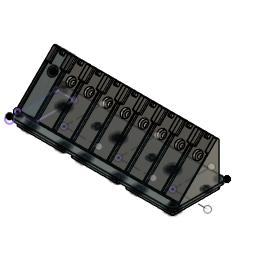
holder_v1 (Autodesk Fusion 360 design; units mm, degrees)
Autodesk Fusion 360 part; units mm, degrees
ref_plane "WorkPlane1" through (12.125, 0, 0) normal (0, -0.707107, 0.707107) x (1, 0, 0) in component "blade_holder"
sketch "Sketch1" plane through (0, 0, 0) normal (0, -0.707107, 0.707107) x (1, 0, 0) in component "blade_holder"
  line L0 (0, 42) -> (14, 42)
  line L1 (14, 42) -> (14, 0)
  line L2 (14, 0) -> (0, 0)
  line L3 (0, 0) -> (0, 42)
  line L4 (1, 41) -> (13, 41)
  line L5 (13, 41) -> (13, 1)
  line L6 (13, 1) -> (1, 1)
  line L7 (1, 1) -> (1, 41)
  line L8 (1, 41) -> (1, 42)
  line L9 (13, 41) -> (13, 42)
  line L10 (6, 42) -> (8, 42)
  line L11 (8, 42) -> (8, 39)
  line L12 (8, 39) -> (6, 39)
  line L13 (6, 39) -> (6, 42)
  line L14 (3, 42) -> (3, 32)
  line L15 (3, 32) -> (1, 32)
  line L16 (11, 42) -> (11, 32)
  line L17 (11, 32) -> (13, 32)
  line L18 (3, 32) -> (11, 32) construction
  circle A0 centre (7, 28.75) radius 3.25
  circle A1 centre (7, 28.75) radius 1.625
  dimension "d7" = 14
  dimension "d8" = 42
  dimension "d9" = 12
  dimension "d10" = 40
  dimension "d11" = 1
  dimension "d12" = 1
  dimension "d14" = 1
  dimension "d15" = 1
  dimension "d22" = 2
  dimension "d23" = 3
  dimension "d24" = 3
  dimension "d25" = 6
  dimension "d40" = 2
  dimension "d41" = 2
  dimension "d42" = 10
  dimension "d43" = 10
  dimension "d116" = 6.5
  dimension "d117" = 6
  dimension "d125" = 3.25
  constraint horizontal L0
  constraint vertical L1
  constraint horizontal L2
  constraint vertical L3
  constraint horizontal L4
  constraint vertical L5
  constraint horizontal L6
  constraint vertical L7
  constraint coincident L0 L8.end
  constraint perpendicular L0 L8
  constraint coincident L0 L9.end
  constraint perpendicular L0 L9
  constraint horizontal L10
  constraint vertical L11
  constraint horizontal L12
  constraint vertical L13
  constraint coincident L0 L14.start
  constraint perpendicular L4 L14
  constraint coincident L7 L15.end
  constraint perpendicular L7 L15
  constraint coincident L0 L16.start
  constraint perpendicular L4 L16
  constraint coincident L5 L17.end
  constraint perpendicular L5 L17
  constraint tangent L18 A0
  constraint concentric A0 A1
  measures "d7" distance of L0.start L0.end
  measures "d8" distance of L0.end L1.end
  measures "d9" distance of L4.start L4.end
  measures "d10" distance of L4.start L6.end
  measures "d11" distance of L0 L4
  measures "d12" distance of L1 L5
  measures "d14" distance of L2.end L6
  measures "d15" distance of L2.end L7
  measures "d22" distance of L10.start L10.end
  measures "d23" distance of L10.end L11.end
  measures "d24" distance of L0 L12
  measures "d25" distance of L3 L13
  measures "d40" distance of L14.end L15.end
  measures "d41" distance of L16.end L17.end
  measures "d42" distance of L16.start L16.end
  measures "d43" distance of L14.start L14.end
  measures "d116" diameter of A0
  measures "d117" distance of L7 A0.centre
  measures "d125" diameter of A1
sketch "Sketch2" plane through (0, 0, 0) normal (0, 0, 1) x (1, 0, 0) in component "blade_holder"
  line L0 (0, 0) -> (0, 29.6985)
  line L1 (0, 29.6985) -> (14, 29.6985)
  line L2 (14, 29.6985) -> (14, 0)
  line L3 (14, 0) -> (0, 0)
sketch "Sketch3" plane through (0, 0, 0) normal (0, 0, 1) x (1, 0, 0) in component "blade_holder"
  line L0 (3.75, 35.8492) -> (122.25, 35.8492)
  line L1 (126, 32.0992) -> (126, -2.4008)
  line L2 (122.25, -6.1508) -> (3.75, -6.1508)
  line L3 (0, -2.4008) -> (0, 32.0992)
  arc A0 (3.75, 35.8492) -> (0, 32.0992) centre (3.75, 32.0992) ccw
  arc A1 (126, 32.0992) -> (122.25, 35.8492) centre (122.25, 32.0992) ccw
  arc A2 (122.25, -6.1508) -> (126, -2.4008) centre (122.25, -2.4008) ccw
  arc A3 (0, -2.4008) -> (3.75, -6.1508) centre (3.75, -2.4008) ccw
  point P0 (0, 35.8492)
  point P1 (126, 35.8492)
  point P2 (0, -6.1508)
  dimension "d91" = 126
  dimension "d92" = 42
  dimension "d93" = 6.1508
  dimension "d95" = 126
  dimension "d96" = 3.75
  dimension "d97" = 3.75
  dimension "d98" = 3.75
  dimension "d99" = 3.75
  constraint horizontal L0
  constraint vertical L1
  constraint horizontal L2
  constraint vertical L3
  constraint coincident P0 L0
  constraint coincident P0 L3
  constraint tangent L0 A0
  constraint tangent L3 A0
  constraint coincident P1 L0
  constraint coincident P1 L1
  constraint tangent L0 A1
  constraint tangent L1 A1
  constraint tangent L1 A2
  constraint tangent L2 A2
  constraint coincident P2 L3
  constraint coincident P2 L2
  constraint tangent L3 A3
  constraint tangent L2 A3
  measures "d91" distance of P0 P1
  measures "d92" distance of P0 P2
  measures "d93" distance of origin L2
  measures "d95" distance of origin L1
  measures "d96" radius of A0
  measures "d97" radius of A1
  measures "d98" radius of A2
  measures "d99" radius of A3
extrude "Extrude1" add sketch "Sketch1" along normal blind 2 contours L0 L1 L2 L3 L5 L6 L7 L8 L9 | L0 L4 L8 L14 | L4 L7 L14 L15 | L0 L4 L9 L16 | L4 L5 L16 L17 makes body 1 in component "blade_holder"
extrude "Extrude2" add sketch "Sketch2" along normal up to surface end surface through (12.125, 0, 0) normal (0, -0.707107, 0.707107) offset 0 bodies 1 in component "blade_holder"
extrude "Extrude3" add sketch "Sketch1" along normal blind 3 contours L0 L4 L10 L11 L13 | L4 L11 L12 L13 bodies 1 in component "blade_holder"
extrude "Extrude7" cut sketch "Sketch1" against normal blind 2.5 contours A0 | A1 bodies 1 in component "blade_holder"
extrude "Extrude8" cut sketch "Sketch1" against normal blind 5 contours A1 bodies 1 in component "blade_holder"
fillet "Fillet1" radius 0.5 8 edges at (6, 28.6378, 30.7591) (6, 26.5165, 30.7591) (7, 27.5772, 31.8198) (8, 28.6378, 30.7591) (8, 26.5165, 30.7591) (7, 25.4558, 29.6985) (8, 26.5165, 28.6378) (6, 26.5165, 28.6378) on bodies 1 in component "blade_holder"
fillet "Fillet1" radius 0.5 17 edges at (3, 28.9914, 30.4056) (3, 21.9203, 23.3345) (1, 10.253, 13.0815) (2, 21.2132, 24.0416) (3, 24.7487, 27.5772) (7, -0.7071, 2.1213) (1, 0, 1.4142) (11, 28.9914, 30.4056) (11, 21.9203, 23.3345) (12, 21.2132, 24.0416) (13, 10.253, 13.0815) (13, 0, 1.4142) (1, 21.9203, 23.3345) (13, 21.9203, 23.3345) (11, 24.7487, 27.5772) (12.5, 28.2843, 31.1127) (1.5, 28.2843, 31.1127) on bodies 1 in component "blade_holder"
extrude "Extrude6" add sketch "Sketch3" against normal blind 2 separate body makes body 2 in component "blade_holder"
sketch "Sketch4" plane through (0, 0, -2) normal (0, 0, -1) x (1, 0, 0) in component "blade_holder"
  arc A0 (0, -32.0992) -> (3.75, -35.8492) centre (3.75, -32.0992) ccw
  line L0 (3.75, -35.8492) -> (122.25, -35.8492)
  arc A1 (122.25, -35.8492) -> (126, -32.0992) centre (122.25, -32.0992) ccw
  line L1 (126, -32.0992) -> (126, 2.4008)
  arc A2 (126, 2.4008) -> (122.25, 6.1508) centre (122.25, 2.4008) ccw
  line L2 (122.25, 6.1508) -> (3.75, 6.1508)
  arc A3 (3.75, 6.1508) -> (0, 2.4008) centre (3.75, 2.4008) ccw
  line L3 (0, 2.4008) -> (0, -32.0992)
  circle A4 centre (8, -1.8492) radius 2.5
  point P0 (0, 6.1508)
  dimension "d104" = 5
  dimension "d105" = 8
  dimension "d106" = 8
  measures "d104" diameter of A4
  measures "d105" vertical distance of A4.centre P0
  measures "d106" horizontal distance of A4.centre P0
pattern_linear "R-Pattern1" count 9 spacing 14 along (1, 0, 0) of bodies 1 makes body 3 at (14, 19.2097, 10.253) makes body 4 at (32.6667, 19.799, 0) makes body 5 at (51.3333, 9.8995, 0) makes body 6 at (60.6667, 19.799, 0) makes body 7 at (74.6667, 19.799, 0) makes body 8 at (88.6667, 19.799, 0) makes body 9 at (102.6667, 19.799, 0) makes body 10 at (126, 19.2097, 10.253) in component "blade_holder"
sketch "Sketch2 (2)" plane through (0, 0, 0) normal (0, 1, 0) x (1, 0, 0) in component "gridfinity_leg"
  line L0 (17.8, 0) -> (18.6, -0.8)
  line L1 (18.6, -0.8) -> (18.6, -2.6)
  line L2 (18.6, -2.6) -> (20.75, -4.75)
  line L3 (0, 0) -> (27.8, 0) construction
  line L4 (20.75, -4.75) -> (0, -4.75)
  line L5 (0, -4.75) -> (0, 0)
  line L6 (17.8, 0) -> (0, 0)
  line L7 (0, -4.75) -> (0, 0)
  dimension "d6_1" = 0.8
  dimension "d7_1" = 45
  dimension "d8_1" = 1.8
  dimension "d9_1" = 2.15
  dimension "d10_1" = 45
  dimension "d15_1" = 20.75
  dimension "d16_1" = 4.75
  constraint vertical L1
  constraint coincident L3.start L5.end
  constraint horizontal L3
  constraint coincident L0.start L3
  constraint perpendicular L3 L5
  measures "d6_1" horizontal distance of L0.start L0.end
  measures "d7_1" angle of L0 L3
  measures "d8_1" distance of L0.end L1.end
  measures "d9_1" horizontal distance of L1.end L2.end
  measures "d10_1" angle of L2 L3
  measures "d15_1" distance of L2.end L4.end
  measures "d16_1" distance of L4.end L3.start
sketch "Sketch4 (2)" plane through (0, 0, 0) normal (0, 0, 1) x (1, 0, 0) in component "gridfinity_leg"
  line L0 (-17, 20.75) -> (17, 20.75)
  line L1 (20.75, 17) -> (20.75, -17)
  line L2 (17, -20.75) -> (-17, -20.75)
  line L3 (-20.75, -17) -> (-20.75, 17)
  arc A0 (-17, 20.75) -> (-20.75, 17) centre (-17, 17) ccw
  arc A1 (20.75, 17) -> (17, 20.75) centre (17, 17) ccw
  arc A2 (17, -20.75) -> (20.75, -17) centre (17, -17) ccw
  arc A3 (-20.75, -17) -> (-17, -20.75) centre (-17, -17) ccw
  point P0 (-20.75, 20.75)
  point P1 (20.75, 20.75)
  point P2 (20.75, -20.75)
  dimension "d43_1" = 41.5
  dimension "d44_1" = 41.5
  dimension "d45_1" = 20.75
  dimension "d46_1" = 20.75
  dimension "d47_1" = 3.75
  dimension "d48_1" = 3.75
  dimension "d49_1" = 3.75
  dimension "d50_1" = 3.75
  constraint horizontal L0
  constraint vertical L1
  constraint horizontal L2
  constraint vertical L3
  constraint coincident P0 L3
  constraint coincident P0 L0
  constraint tangent L3 A0
  constraint tangent L0 A0
  constraint coincident P1 L0
  constraint coincident P1 L1
  constraint tangent L0 A1
  constraint tangent L1 A1
  constraint coincident P2 L1
  constraint coincident P2 L2
  constraint tangent L1 A2
  constraint tangent L2 A2
  constraint tangent L3 A3
  constraint tangent L2 A3
  measures "d43_1" distance of P0 P1
  measures "d44_1" distance of P1 P2
  measures "d45_1" distance of L0 origin
  measures "d46_1" distance of L3 origin
  measures "d47_1" radius of A0
  measures "d48_1" radius of A1
  measures "d49_1" radius of A2
  measures "d50_1" radius of A3
sketch "Sketch5" plane through (0, 0, 0) normal (0, 0, 1) x (1, 0, 0) in component "gridfinity_leg"
  circle A0 centre (13, 13) radius 3.25
  circle A1 centre (13, 13) radius 1.5
  line L0 (0, 0) -> (0, 30) construction
  line L1 (0, 0) -> (27, 0) construction
  line L2 (11.5, 15.8831) -> (11.5, 10.1169)
  line L3 (14.5, 15.8831) -> (14.5, 10.1169)
  line L4 (10.1169, 11.5) -> (15.8831, 11.5)
  line L5 (10.1169, 14.5) -> (15.8831, 14.5)
  line L6 (-10.1169, 11.5) -> (-15.8831, 11.5)
  circle A2 centre (-13, 13) radius 3.25
  line L7 (-14.5, 15.8831) -> (-14.5, 10.1169)
  line L8 (-10.1169, 14.5) -> (-15.8831, 14.5)
  line L9 (-11.5, 15.8831) -> (-11.5, 10.1169)
  circle A3 centre (-13, 13) radius 1.5
  line L10 (10.1169, -11.5) -> (15.8831, -11.5)
  line L11 (11.5, -15.8831) -> (11.5, -10.1169)
  line L12 (10.1169, -14.5) -> (15.8831, -14.5)
  line L13 (14.5, -15.8831) -> (14.5, -10.1169)
  circle A4 centre (13, -13) radius 3.25
  circle A5 centre (13, -13) radius 1.5
  circle A6 centre (-13, -13) radius 3.25
  line L14 (-10.1169, -14.5) -> (-15.8831, -14.5)
  line L15 (-14.5, -15.8831) -> (-14.5, -10.1169)
  line L16 (-11.5, -15.8831) -> (-11.5, -10.1169)
  line L17 (-10.1169, -11.5) -> (-15.8831, -11.5)
  circle A7 centre (-13, -13) radius 1.5
  dimension "d57_1" = 6.5
  dimension "d58_1" = 3
  dimension "d59_1" = 13
  dimension "d60_1" = 13
  dimension "d61_1" = 3
  dimension "d62_1" = 3
  constraint concentric A0 A1
  constraint coincident L0.start L1.start
  constraint vertical L0
  constraint perpendicular L0 L1
  constraint coincident A0 L2.start
  constraint coincident A0 L2.end
  constraint vertical L2
  constraint coincident A0 L3.start
  constraint coincident A0 L3.end
  constraint parallel L2 L3
  constraint coincident A0 L4.start
  constraint coincident A0 L4.end
  constraint perpendicular L3 L4
  constraint coincident A0 L5.start
  constraint coincident A0 L5.end
  constraint perpendicular L3 L5
  constraint tangent A1 L5
  constraint tangent A1 L3
  constraint symmetric A0 L0 A2
  constraint symmetric A1 L0 A3
  constraint symmetric L0 L2.start L9.start
  constraint symmetric L0 L2.end L9.end
  constraint symmetric L0 L3.start L7.start
  constraint symmetric L0 L3.end L7.end
  constraint symmetric L0 L4.start L6.start
  constraint symmetric L0 L4.end L6.end
  constraint symmetric L0 L5.start L8.start
  constraint symmetric L0 L5.end L8.end
  constraint symmetric A0 L1 A4
  constraint symmetric A1 L1 A5
  constraint symmetric L1 L2.start L11.start
  constraint symmetric L1 L2.end L11.end
  constraint symmetric L1 L3.start L13.start
  constraint symmetric L1 L3.end L13.end
  constraint symmetric L1 L4.start L10.start
  constraint symmetric L1 L4.end L10.end
  constraint symmetric L1 L5.start L12.start
  constraint symmetric L1 L5.end L12.end
  constraint symmetric L1 L9.end L16.end
  constraint symmetric L1 L9.start L16.start
  constraint symmetric L1 L7.start L15.start
  constraint symmetric L1 L8.end L14.end
  constraint symmetric L1 L6.start L17.start
  constraint symmetric L1 L6.end L17.end
  constraint symmetric L1 L8.start L14.start
  constraint symmetric L1 L7.end L15.end
  constraint symmetric L1 A2 A6
  constraint symmetric L1 A3 A7
  measures "d57_1" diameter of A0
  measures "d58_1" diameter of A1
  measures "d59_1" vertical distance of L0.start A0.centre
  measures "d60_1" horizontal distance of L0.start A0.centre
  measures "d61_1" distance of L4 L5
  measures "d62_1" distance of L2 L3
sweep "Sweep1" add profiles "Sketch2 (2)" path "Sketch4 (2)" along A2 L2 A3 L3 A0 L0 A1 L1 section 1 separate body makes body 11 in component "gridfinity_leg"
extrude "Extrude4" cut sketch "Sketch5" along normal blind 2.4 bodies 11 in component "gridfinity_leg"
extrude "Extrude5" cut sketch "Sketch5" along normal blind 0.2 from surface at 2.4 contours A0 L3 L4 L5 | A1 L3 L5 | A1 L3 L4 | A1 L2 L5 | A1 L2 L4 | A0 L2 L4 L5 | L6 A2 L8 L9 | L6 L9 A3 | L6 L7 A3 | L8 L9 A3 | L6 A2 L7 L8 | L7 L8 A3 | L10 L11 L12 A4 | L10 L11 A5 | L10 L13 A5 | L11 L12 A5 | L10 L12 L13 A4 | L12 L13 A5 | A6 L14 L16 L17 | L16 L17 A7 | L14 L16 A7 | L15 L17 A7 | L14 L15 A7 | A6 L14 L15 L17 bodies 11 in component "gridfinity_leg"
extrude "Extrude6'" cut sketch "Sketch5" along normal blind 0.4 from surface at 2.4 contours A1 L3 L5 | A1 L3 L4 | A1 L2 L5 | A1 L2 L4 | L6 L9 A3 | L6 L7 A3 | L8 L9 A3 | L7 L8 A3 | L10 L11 A5 | L10 L13 A5 | L11 L12 A5 | L12 L13 A5 | L16 L17 A7 | L14 L16 A7 | L15 L17 A7 | L14 L15 A7 bodies 11 in component "gridfinity_leg"
extrude "Extrude7'" cut sketch "Sketch5" along normal blind 10 contours A1 | A3 | A5 | A7 bodies 11 in component "gridfinity_leg"
pattern_linear "00000000-0000-0000-0000-000000000000" [suppressed]
component "blade_holder" placed x (1, 0, 0) y (0, 1, 0) z (0, 0, 1) at (-21, -14.8492, 6.75)
component "gridfinity_leg" placed x (1, 0, 0) y (0, 1, 0) z (0, 0, 1) at (0, 0, 0)
component "gridfinity_leg" placed x (1, 0, 0) y (0, 1, 0) z (0, 0, 1) at (42, 0, 0)
component "gridfinity_leg" placed x (1, 0, 0) y (0, 1, 0) z (0, 0, 1) at (84, 0, 0)
equation "edit_blade_height = 40 mm"
equation "edit_blade_width = 12 mm"
equation "gridfinity_outer_size = 42 mm"
equation "d4 = blade_holder_angle"
equation "blade_holder_angle = 45 deg"
equation "blade_holder_border_width = 1 mm"
equation "d7 = edit_blade_width + 2 * blade_holder_border_width"
equation "d8 = edit_blade_height + 2 * blade_holder_border_width"
equation "d9 = edit_blade_width"
equation "d10 = edit_blade_height"
equation "d11 = blade_holder_border_width"
equation "d12 = blade_holder_border_width"
equation "d14 = blade_holder_border_width"
equation "d15 = blade_holder_border_width"
equation "d16 = blade_holder_border_height"
equation "blade_hook_height = 3 mm"
equation "blade_hook_width = 2 mm"
equation "d22 = blade_hook_width"
equation "d23 = blade_hook_height"
equation "d24 = blade_hook_height"
equation "d25 = ( edit_blade_width + 2 * blade_holder_border_width ) / 2 - blade_hook_width / 2"
equation "blade_hook_depth = 3 mm"
equation "blade_hook_fillet = max(0.5 mm; blade_holder_border_width / 2)"
equation "d28 = blade_hook_depth"
equation "d31 = blade_hook_fillet"
equation "blade_side_holder_height = 10 mm"
equation "blade_side_holder_width = 2 mm"
equation "d40 = blade_side_holder_width"
equation "d41 = blade_side_holder_width"
equation "d42 = blade_side_holder_height"
equation "d43 = blade_side_holder_height"
equation "edit_blade_holder_magnet_depth = 2.5 mm"
equation "edit_blade_holder_count = 9"
equation "blade_holder_leg_size = ceil(( edit_blade_width + 2 * blade_holder_border_width ) * edit_blade_holder_count / gridfinity_outer_size) * gridfinity_outer_size"
equation "blade_holder_leg_height = 2 mm"
equation "d80 = -blade_holder_leg_height"
equation "blade_holder_width = cos(blade_holder_angle) * ( edit_blade_height + 2 * blade_holder_border_width )"
equation "d91 = blade_holder_leg_size"
equation "d92 = gridfinity_outer_size"
equation "d93 = ( gridfinity_outer_size - blade_holder_width ) / 2"
equation "d95 = blade_holder_leg_size - ( blade_holder_leg_size - ( ( edit_blade_width + 2 * blade_holder_border_width ) * edit_blade_holder_count ) ) / 2"
equation "d100 = edit_blade_holder_count"
equation "d102 = edit_blade_width + blade_holder_border_width * 2"
equation "d45_1 = ( 41.5 / 2 ) * 1 mm"
equation "d46_1 = ( 41.5 / 2 ) * 1 mm"
equation "d47_1 = ( 7.5 / 2 ) * 1 mm"
equation "d48_1 = ( 7.5 / 2 ) * 1 mm"
equation "d49_1 = ( 7.5 / 2 ) * 1 mm"
equation "d50_1 = ( 7.5 / 2 ) * 1 mm"
equation "d67_1 = print_layer_height"
equation "d70_1 = print_layer_height * 2"
equation "print_layer_height = 0.2 mm"
equation "d111 = blade_holder_leg_size / gridfinity_outer_size"
equation "d113 = gridfinity_outer_size"
equation "edit_blade_magnet_diameter = 6.5 mm"
equation "d116 = edit_blade_magnet_diameter"
equation "d117 = edit_blade_width / 2"
equation "d118 = -edit_blade_holder_magnet_depth"
equation "blade_holder_border_height = 2 mm"
equation "d124 = blade_hook_fillet"
equation "d125 = edit_blade_magnet_diameter / 2"
equation "d126 = -2 * edit_blade_holder_magnet_depth"
